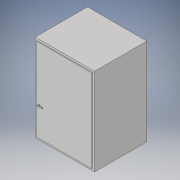
# Autodesk Inventor part: enclosureNode
Saved by Autodesk Inventor 2017 (Build 210142000, 142)
## iProperties
Created: 2016-06-20
Part Number: enclosureNode
Material: Generic
Document SubType Name: Modeling
Designer: Zuhra Abdurashidova
Density: 1 g/cm^3
Appearance: Default
Author: Zuhra Abdurashidova
Autodesk Inventor part; units mm, degrees
ref_plane "YZ Plane" through (0, 0, 0) normal (1, 0, 0) x (0, 1, 0)
ref_plane "XZ Plane" through (0, 0, 0) normal (0, 1, 0) x (-1, 0, 0)
ref_plane "XY Plane" through (0, 0, 0) normal (0, 0, 1) x (1, 0, 0)
sketch "Sketch1" plane through (0, 0, 0) normal (0, 1, 0) x (-1, 0, 0)
  point P0 (0, 0)
sketch "Sketch2" plane through (0, 0, 0) normal (0, 1, 0) x (-1, 0, 0)
  line L0 (-432, 381) -> (432, 381)
  line L1 (432, 381) -> (432, -381)
  line L2 (432, -381) -> (-432, -381)
  line L3 (-432, -381) -> (-432, 381)
  line L4 (-432, 381) -> (432, -381) construction
  line L5 (432, 381) -> (-432, -381) construction
  point P0 (0, 0)
  dimension "d16" = 762
  dimension "d17" = 864
  constraints: 12 end point, 2 midpoint, 2 parallel, 1 horizontal, 1 perpendicular
  measures "d16" distance of L0.end L1.end
  measures "d17" distance of L1.end L2.end
extrude "Node" add sketch "Sketch2" along normal blind 1270
shell "Shell1" thickness 30 removed faces 0
sketch "Sketch3" plane through (-432, 0, 381) normal (0, 0, 1) x (1, 0, 0)
  line L0 (30, 30) -> (834, 30)
  line L1 (834, 30) -> (834, 1240)
  line L2 (834, 1240) -> (30, 1240)
  line L3 (30, 1240) -> (30, 30)
  line L4 (30, 30) -> (834, 1240) construction
  line L5 (834, 30) -> (30, 1240) construction
  line L6 (864, 0) -> (864, 1270) projected
  line L7 (0, 1270) -> (864, 1270) projected
  line L8 (0, 0) -> (0, 1270) projected
  line L9 (864, 0) -> (0, 0) projected
  point P0 (432, 0)
  point P1 (432, 635)
  dimension "d21" = 30
  dimension "d22" = 30
  dimension "d23" = 30
  dimension "d24" = 30
  constraints: 12 end point, 2 midpoint, 2 parallel, 1 horizontal, 1 perpendicular
  measures "d21" distance between parallel lines of L6 L1
  measures "d22" distance between parallel lines of L7 L2
  measures "d23" distance between parallel lines of L8 L3
  measures "d24" distance between parallel lines of L9 L0
extrude "Door" add sketch "Sketch3" along normal blind 10 contours L3 L2 L1 L0
sketch "Sketch5" plane through (-432, 0, 391) normal (0, 0, 1) x (1, 0, 0)
  line L0 (59.5914, 457.1317) -> (79.5601, 457.1317)
  line L1 (79.5601, 457.1317) -> (79.5601, 442.8683)
  line L2 (79.5601, 442.8683) -> (59.5914, 442.8683)
  line L3 (59.5914, 442.8683) -> (59.5914, 457.1317)
  line L4 (59.5914, 457.1317) -> (79.5601, 442.8683) construction
  line L5 (79.5601, 457.1317) -> (59.5914, 442.8683) construction
  point P0 (432, 0)
  point P1 (69.5757, 450)
  constraints: 12 end point, 2 midpoint, 2 parallel, 1 horizontal, 1 perpendicular
extrude "handle1" add sketch "Sketch5" along normal blind 20
sketch "Sketch6" plane through (-352.4399, 442.8683, 391) normal (1, 0, 0) x (0, 0, -1)
  line L0 (-20, 14.2634) -> (-12.9022, 14.2634)
  line L1 (-12.9022, 14.2634) -> (-12.9022, -0.0578)
  line L2 (-12.9022, -0.0578) -> (-20, -0.0578)
  line L3 (-20, -0.0578) -> (-20, 14.2634)
  point P0 (391, -442.8683)
  constraints: 8 end point, 2 parallel, 1 horizontal, 1 perpendicular
extrude "handle2" add sketch "Sketch6" along normal blind 50
body "Solid2"
